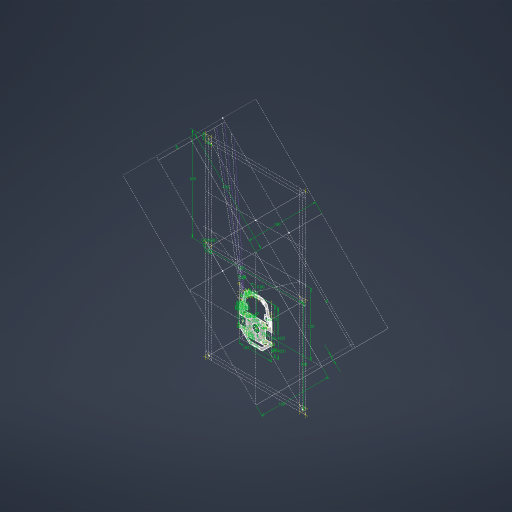
# Autodesk Inventor part: chassis
Saved by Autodesk Inventor 2023.5 (Build 275446000, 446)
## iProperties
Created: 2024-12-08
Part Number: chassis
Material: 一般
Document SubType Name: Modeling
Designer: IshiiLabHonda
Density: 1 g/cm^3
Appearance: 既定
Author: IshiiLabHonda
Autodesk Inventor part; units mm, degrees
(part 1 of 2)
ref_plane "YZ Plane" through (0, 0, 0) normal (1, 0, 0) x (0, 1, 0)
ref_plane "XZ Plane" through (0, 0, 0) normal (0, 1, 0) x (-1, 0, 0)
ref_plane "XY Plane" through (0, 0, 0) normal (0, 0, 1) x (1, 0, 0)
sketch "スケッチ1" plane through (0, 0, 0) normal (0, 0, 1) x (1, 0, 0)
  line L0 (0, 0) -> (0, 1) construction
  line L1 (0, 0) -> (1, 0) construction
  line L2 (-90, 90) -> (90, 90) construction
  line L3 (90, 90) -> (90, -90) construction
  line L4 (90, -90) -> (-90, -90) construction
  line L5 (-90, -90) -> (-90, 90) construction
  line L6 (-90, -90) -> (90, 90) construction
  line L7 (-90, 90) -> (90, -90) construction
  line L8 (-84, 96) -> (-84, 84) construction
  line L9 (-84, 84) -> (-96, 84) construction
  line L10 (-96, 84) -> (-96, 96) construction
  line L11 (-96, 96) -> (-84, 84) construction
  line L12 (-84, 96) -> (-96, 84) construction
  line L13 (-96, 96) -> (-84, 96) construction
  line L14 (-96, -96) -> (-96, -84) construction
  line L15 (-84, -96) -> (-96, -96) construction
  line L16 (-96, -96) -> (-84, -84) construction
  line L17 (-96, -84) -> (-84, -96) construction
  line L18 (-84, -84) -> (-84, -96) construction
  line L19 (-96, -84) -> (-84, -84) construction
  line L20 (96, -96) -> (84, -96) construction
  line L21 (96, -84) -> (96, -96) construction
  line L22 (96, -96) -> (84, -84) construction
  line L23 (84, -96) -> (96, -84) construction
  line L24 (84, -84) -> (96, -84) construction
  line L25 (84, -96) -> (84, -84) construction
  line L26 (96, 96) -> (96, 84) construction
  line L27 (84, 96) -> (96, 96) construction
  line L28 (96, 96) -> (84, 84) construction
  line L29 (96, 84) -> (84, 96) construction
  line L30 (84, 84) -> (84, 96) construction
  line L31 (96, 84) -> (84, 84) construction
  line L32 (-84, 84) -> (-84, -84) construction
  line L33 (-96, 84) -> (-96, -84) construction
  line L34 (-84, -84) -> (84, -84) construction
  line L35 (-84, -96) -> (84, -96) construction
  line L36 (96, 84) -> (96, -84) construction
  line L37 (84, 84) -> (84, -84) construction
  line L38 (-84, 96) -> (84, 96) construction
  line L39 (-84, 84) -> (84, 84) construction
  line L40 (-19, 15) -> (19, 15) construction
  line L41 (19, 15) -> (19, -15) construction
  line L42 (19, -15) -> (-19, -15) construction
  line L43 (-19, -15) -> (-19, 15) construction
  line L44 (-19, 15) -> (19, -15) construction
  line L45 (19, 15) -> (-19, -15) construction
  line L46 (-30.25, 11.5) -> (-19, 11.5) construction
  line L47 (-19, -11.5) -> (-30.25, -11.5) construction
  line L48 (-30.25, -11.5) -> (-30.25, 11.5) construction
  line L49 (-30.25, 11.5) -> (-19, -11.5) construction
  line L50 (-19, 11.5) -> (-30.25, -11.5) construction
  line L51 (30.25, 11.5) -> (19, 11.5) construction
  line L52 (19, -11.5) -> (30.25, -11.5) construction
  line L53 (30.25, -11.5) -> (30.25, 11.5) construction
  line L54 (30.25, 11.5) -> (19, -11.5) construction
  line L55 (19, 11.5) -> (30.25, -11.5) construction
  line L56 (-19, -10) -> (19, -10) construction
  line L57 (-19, -12.5) -> (19, -12.5) construction
  line L58 (-19, 10) -> (19, 10) construction
  line L59 (-19, 12.5) -> (19, 12.5) construction
  line L60 (-16.5, -15) -> (-16.5, 15) construction
  line L61 (16.5, -15) -> (16.5, 15) construction
  line L62 (-12.5, -10) -> (-12.5, -15) construction
  line L63 (-16.5, -10) -> (-12.5, -15) construction
  line L64 (-16.5, -15) -> (-12.5, -10) construction
  circle A0 centre (-14.5, -12.5) radius 0.8 construction
  line L65 (12.5, -10) -> (12.5, -15) construction
  line L66 (16.5, -10) -> (12.5, -15) construction
  line L67 (16.5, -15) -> (12.5, -10) construction
  circle A1 centre (14.5, -12.5) radius 0.8 construction
  line L68 (-12.5, 10) -> (-12.5, 15) construction
  line L69 (-16.5, 10) -> (-12.5, 15) construction
  line L70 (-16.5, 15) -> (-12.5, 10) construction
  circle A2 centre (-14.5, 12.5) radius 0.8 construction
  line L71 (12.5, 10) -> (12.5, 15) construction
  line L72 (16.5, 10) -> (12.5, 15) construction
  circle A3 centre (14.5, 12.5) radius 0.8 construction
  line L73 (16.5, 15) -> (12.5, 10) construction
  line L74 (-96, 276) -> (-84, 276) construction
  line L75 (-84, 276) -> (-84, 264) construction
  line L76 (-84, 264) -> (-96, 264) construction
  line L77 (-96, 264) -> (-96, 276) construction
  line L78 (-96, 276) -> (-84, 264) construction
  line L79 (-84, 276) -> (-96, 264) construction
  line L80 (-90, 90) -> (-90, 270) construction
  line L81 (-96, 264) -> (-96, 96) construction
  line L82 (-84, 264) -> (-84, 96) construction
  line L83 (96, 276) -> (84, 276) construction
  line L84 (84, 276) -> (84, 264) construction
  line L85 (84, 264) -> (96, 264) construction
  line L86 (96, 264) -> (96, 276) construction
  line L87 (96, 276) -> (84, 264) construction
  line L88 (84, 276) -> (96, 264) construction
  line L89 (90, 90) -> (90, 270) construction
  line L90 (96, 264) -> (96, 96) construction
  line L91 (84, 264) -> (84, 96) construction
  line L92 (-84, 276) -> (84, 276) construction
  line L93 (-84, 264) -> (84, 264) construction
  line L94 (-90, 270) -> (90, 270) construction
  line L95 (-90, 270) -> (90, 90) construction
  line L96 (-90, 90) -> (90, 270) construction
  circle A4 centre (0, 0) radius 15 construction
  line L97 (-96, 120) -> (96, 120) construction
  line L98 (0, 127.279221) -> (0, -127.279221) construction
  line L99 (-127.279221, 0) -> (127.279221, 0) construction
  line L100 (127.279221, 0) -> (0, -127.279221) construction
  line L101 (0, -127.279221) -> (-127.279221, 0) construction
  line L102 (-127.279221, 0) -> (0, 127.279221) construction
  line L103 (0, 127.279221) -> (127.279221, 0) construction
  line L104 (127.279221, 254.558441) -> (254.558441, 127.279221) construction
  line L105 (254.558441, 127.279221) -> (127.279221, 0) construction
  line L106 (127.279221, 0) -> (0, 127.279221) construction
  line L107 (0, 127.279221) -> (127.279221, 254.558441) construction
  line L108 (-127.279221, 254.558441) -> (0, 127.279221) construction
  line L109 (0, 127.279221) -> (-127.279221, 0) construction
  line L110 (-127.279221, 0) -> (-254.558441, 127.279221) construction
  line L111 (-254.558441, 127.279221) -> (-127.279221, 254.558441) construction
  line L112 (0, 381.837662) -> (127.279221, 254.558441) construction
  line L113 (127.279221, 254.558441) -> (0, 127.279221) construction
  line L114 (0, 127.279221) -> (-127.279221, 254.558441) construction
  line L115 (-127.279221, 254.558441) -> (0, 381.837662) construction
  line L116 (190.918831, 63.63961) -> (63.63961, 190.918831) construction
  line L117 (-190.918831, 190.918831) -> (-63.63961, 63.63961) construction
  line L118 (59.39697, -59.39697) -> (186.67619, 67.882251) construction
  line L119 (59.39697, 186.67619) -> (186.67619, 59.39697) construction
  line L120 (63.63961, 190.918831) -> (-63.63961, 318.198052) construction
  line L121 (-186.67619, 186.67619) -> (-59.39697, 313.955411) construction
  point P0 (-90, -90)
  point P1 (90, -90)
  point P2 (-24.625, 0)
  point P3 (-84, 120)
  point P4 (84, 120)
  point P5 (0, 0)
  dimension "d0" = 1
  dimension "d1" = 1
  dimension "d2" = 180
  dimension "d3" = 180
  dimension "d4" = 12
  dimension "d5" = 12
  dimension "d8" = 360
  dimension "d10" = 38
  dimension "d12" = 11.25
  dimension "d13" = 23
  dimension "d14" = 5
  dimension "d15" = 2.5
  dimension "d16" = 4
  dimension "d17" = 1.6
  dimension "d22" = 12
  dimension "d23" = 12
  dimension "d24" = 180
  dimension "d25" = 25
  dimension "d26" = 30
  dimension "d27" = 30
  dimension "d29" = 120
  dimension "d331" = 180
  dimension "d334" = 180
  dimension "d337" = 180
  dimension "d340" = 6
  dimension "d341" = 6
  dimension "d342" = 6
  dimension "d561" = 33
  constraints: 244 end point, 29 point on line, 27 symmetric about line, 19 midpoint, 18 parallel, 10 perpendicular, 5 centre point, 4 coincident, 2 collinear, 1 horizontal, 1 vertical, 91 other
  measures "d0" distance of L0.start L0.end
  measures "d1" distance of L0.start L1.end
  measures "d2" distance of L2.start L2.end
  measures "d3" distance of L2.end L3.end
  measures "d4" distance of L9.end L10.end
  measures "d5" distance of L8.end L9.end
  measures "d10" distance of L40.start L40.end
  measures "d12" distance of L46.start L46.end
  measures "d13" distance of L47.end L46.start
  measures "d14" distance between parallel lines of L56 L42
  measures "d15" distance between parallel lines of L43 L60
  measures "d16" distance between parallel lines of L60 L62
  measures "d17" diameter of A0
  measures "d22" distance of L75.end L76.end
  measures "d23" distance of L76.end L74.start
  measures "d24" distance of L2.start L80.end
  measures "d25" distance between parallel lines of L57 L59
  measures "d26" distance between parallel lines of L42 L40
  measures "d27" diameter of A4
  measures "d29" distance between parallel lines of L1 L97
  measures "d331" distance of L100.start L100.end
  measures "d334" distance of L102.end L104.start
  measures "d337" distance of L102.end L108.start
  measures "d340" distance between parallel lines of L118 L105
  measures "d341" distance between parallel lines of L116 L119
  measures "d342" distance between parallel lines of L111 L121
  measures "d561" distance between parallel lines of L61 L60
sketch "スケッチ4" plane through (0, 0, 0) normal (0, 0, 1) x (1, 0, 0)
  line L0 (-84, 264) -> (-96, 264) construction
  line L1 (-90, 90) -> (-90, 270) construction
  line L2 (-96, 264) -> (-96, 96) construction
  line L3 (-96, 96) -> (-84, 96) construction
  line L4 (-84, 96) -> (-84, 84) construction
  line L5 (-84, 96) -> (-96, 84) construction
  line L6 (-96, 96) -> (-84, 84) construction
  line L7 (-84, 264) -> (-84, 96) construction
  line L8 (-84, 84) -> (-96, 84) construction
  line L9 (84, -84) -> (96, -84) construction
  line L10 (84, -96) -> (96, -84) construction
  line L11 (96, -96) -> (84, -84) construction
  line L12 (96, -84) -> (96, -96) construction
  line L13 (96, -96) -> (84, -96) construction
  line L14 (0, 0) -> (0, 1) construction
  line L15 (0, 0) -> (1, 0) construction
  line L16 (16.5, 15) -> (12.5, 10) construction
  line L17 (-96, 84) -> (-96, -84) construction
  line L18 (-84, 84) -> (-84, -84) construction
  line L19 (-90, -90) -> (-90, 90) construction
  line L20 (-90, 90) -> (90, 90) construction
  line L21 (-84, -84) -> (84, -84) construction
  line L22 (-84, -96) -> (84, -96) construction
  line L23 (-90, -90) -> (90, 90) construction
  line L24 (90, -90) -> (-90, -90) construction
  line L25 (-90, 90) -> (90, -90) construction
  line L26 (84, 84) -> (84, -84) construction
  line L27 (90, 90) -> (90, -90) construction
  line L28 (96, 84) -> (96, -84) construction
  line L29 (-96, 84) -> (-96, 96) construction
  line L30 (-84, -84) -> (-84, -96) construction
  line L31 (-96, -84) -> (-84, -84) construction
  line L32 (-84, -96) -> (-96, -96) construction
  line L33 (-96, -96) -> (-84, -84) construction
  line L34 (-96, -84) -> (-84, -96) construction
  line L35 (-96, -96) -> (-96, -84) construction
  line L36 (84, -96) -> (84, -84) construction
  line L37 (-19, -15) -> (-19, 15) construction
  line L38 (-30.25, 11.5) -> (-19, 11.5) construction
  line L39 (-19, -11.5) -> (-30.25, -11.5) construction
  line L40 (-19, 11.5) -> (-30.25, -11.5) construction
  line L41 (-30.25, 11.5) -> (-19, -11.5) construction
  line L42 (-30.25, -11.5) -> (-30.25, 11.5) construction
  line L43 (12.5, 10) -> (12.5, 15) construction
  circle A0 centre (14.5, 12.5) radius 0.8 construction
  line L44 (30.25, 11.5) -> (19, 11.5) construction
  line L45 (16.5, 10) -> (12.5, 15) construction
  circle A1 centre (14.5, -12.5) radius 0.8 construction
  line L46 (16.5, -15) -> (12.5, -10) construction
  line L47 (16.5, -10) -> (12.5, -15) construction
  line L48 (12.5, -10) -> (12.5, -15) construction
  circle A2 centre (-14.5, -12.5) radius 0.8 construction
  line L49 (-12.5, -10) -> (-12.5, -15) construction
  line L50 (-16.5, -15) -> (-12.5, -10) construction
  line L51 (-16.5, -10) -> (-12.5, -15) construction
  line L52 (96, 84) -> (84, 84) construction
  line L53 (96, 96) -> (96, 84) construction
  line L54 (84, 96) -> (96, 96) construction
  line L55 (96, 96) -> (84, 84) construction
  line L56 (84, 84) -> (84, 96) construction
  line L57 (96, 84) -> (84, 96) construction
  line L58 (-96, 264) -> (-96, 276) construction
  line L59 (-84, 276) -> (-84, 264) construction
  line L60 (-96, 276) -> (-84, 276) construction
  line L61 (-96, 276) -> (-84, 264) construction
  line L62 (-84, 276) -> (-96, 264) construction
  line L63 (-84, 84) -> (84, 84) construction
  line L64 (-84, 96) -> (84, 96) construction
  line L65 (84, 264) -> (84, 96) construction
  line L66 (90, 90) -> (90, 270) construction
  line L67 (-90, 90) -> (90, 270) construction
  line L68 (-90, 270) -> (90, 90) construction
  line L69 (96, 264) -> (96, 96) construction
  line L70 (-96, 120) -> (96, 120) construction
  line L71 (-84, 264) -> (84, 264) construction
  line L72 (-84, 276) -> (84, 276) construction
  line L73 (-90, 270) -> (90, 270) construction
  line L74 (84, 276) -> (84, 264) construction
  line L75 (84, 264) -> (96, 264) construction
  line L76 (96, 264) -> (96, 276) construction
  line L77 (96, 276) -> (84, 264) construction
  line L78 (96, 276) -> (84, 276) construction
  line L79 (84, 276) -> (96, 264) construction
  line L80 (-19, 15) -> (19, 15) construction
  line L81 (19, 15) -> (19, -15) construction
  line L82 (19, -15) -> (-19, -15) construction
  circle A3 centre (-14.5, 12.5) radius 0.8 construction
  line L83 (-16.5, 10) -> (-12.5, 15) construction
  line L84 (-12.5, 10) -> (-12.5, 15) construction
  line L85 (-16.5, 15) -> (-12.5, 10) construction
  circle A4 centre (0, 0) radius 15 construction
  line L86 (-19, 10) -> (19, 10) construction
  line L87 (-19, 12.5) -> (19, 12.5) construction
  line L88 (-19, 15) -> (19, -15) construction
  line L89 (19, 15) -> (-19, -15) construction
  line L90 (-19, -10) -> (19, -10) construction
  line L91 (-19, -12.5) -> (19, -12.5) construction
  line L92 (16.5, -15) -> (16.5, 15) construction
  line L93 (19, 11.5) -> (30.25, -11.5) construction
  line L94 (19, -11.5) -> (30.25, -11.5) construction
  line L95 (30.25, -11.5) -> (30.25, 11.5) construction
  line L96 (30.25, 11.5) -> (19, -11.5) construction
  line L97 (-16.5, -15) -> (-16.5, 15) construction
  line L98 (-84, 120) -> (30.25, 40.001289) construction
  line L99 (84, 120) -> (-30.25, 40.001289) construction
  line L100 (-30.25, 57) -> (30.25, 57) construction
  line L101 (1.000463, 57) -> (-30.25, 35.11819) construction
  line L102 (-1.000463, 57) -> (30.25, 35.11819) construction
  line L103 (-12.947112, 57) -> (-30.25, 44.884387) construction
  line L104 (-14.32927, 55.421815) -> (-10.314235, 49.68775) construction
  line L105 (-10.314235, 49.68775) -> (-15.638724, 45.959504) construction
  line L106 (-15.638724, 45.959504) -> (-19.653759, 51.693568) construction
  line L107 (-19.653759, 51.693568) -> (-14.32927, 55.421815) construction
  line L108 (-14.32927, 55.421815) -> (-15.638724, 45.959504) construction
  line L109 (-10.314235, 49.68775) -> (-19.653759, 51.693568) construction
  line L110 (-13.755694, 54.602663) -> (-19.080182, 50.874416) construction
  line L111 (-10.887812, 50.506903) -> (-16.2123, 46.778656) construction
  line L112 (-14.983997, 50.690659) -> (-14.328675, 51.14952) construction
  line L113 (-14.983997, 50.690659) -> (-14.525136, 50.035338) construction
  line L114 (-14.615634, 52.779752) -> (-12.894904, 50.322296) construction
  line L115 (-12.894904, 50.322296) -> (-15.35236, 48.601566) construction
  line L116 (-15.35236, 48.601566) -> (-17.07309, 51.059023) construction
  line L117 (-17.07309, 51.059023) -> (-14.615634, 52.779752) construction
  line L118 (-14.615634, 52.779752) -> (-15.35236, 48.601566) construction
  line L119 (-12.894904, 50.322296) -> (-17.07309, 51.059023) construction
  circle A5 centre (-14.983997, 50.690659) radius 0.8 construction
  line L120 (-30.25, 11.5) -> (-30.25, 57) construction
  line L121 (30.25, 11.5) -> (30.25, 57) construction
  line L122 (-6.140277, 52) -> (6.140277, 52) construction
  line L123 (-31, 57) -> (-31, -31) construction
  line L124 (31, 57) -> (31, -31) construction
  line L125 (-30.25, 57) -> (-31, 57) construction
  line L126 (30.25, 57) -> (31, 57) construction
  line L127 (-31, 8.5) -> (31, 8.5) construction
  line L128 (-31, -8.5) -> (31, -8.5) construction
  circle A6 centre (0, 0) radius 7.5 construction
  line L129 (-31, -31) -> (31, -31) construction
  line L130 (-30.25, 44.884387) -> (-31, 44.359231) construction
  line L131 (-30.25, 35.11819) -> (-31, 34.593035) construction
  line L132 (-25.25, 26.5) -> (-25.361338, 27.292214) construction
  line L133 (-25.25, 26.5) -> (-24.457786, 26.611338) construction
  line L134 (-28.073603, 28.627737) -> (-23.122263, 29.323603) construction
  line L135 (-23.122263, 29.323603) -> (-22.426397, 24.372263) construction
  line L136 (-22.426397, 24.372263) -> (-27.377737, 23.676397) construction
  line L137 (-27.377737, 23.676397) -> (-28.073603, 28.627737) construction
  line L138 (-28.073603, 28.627737) -> (-22.426397, 24.372263) construction
  line L139 (-23.122263, 29.323603) -> (-27.377737, 23.676397) construction
  circle A7 centre (-25.25, 26.5) radius 0.8 construction
  line L140 (-25.25, 57) -> (-25.25, -31) construction
  line L141 (-96, 180) -> (96, 180) construction
  line L142 (-25.361338, 27.292214) -> (-64.878802, 308.473578) construction
  line L143 (-186.67619, 186.67619) -> (-59.39697, 313.955411) construction
  line L144 (59.39697, 186.67619) -> (186.67619, 59.39697) construction
  line L145 (-25.25, 26.5) -> (-79.619204, 293.733176) construction
  line L146 (-25.25, 26.5) -> (-46.888819, 301.44726) construction
  line L147 (63.63961, 190.918831) -> (-63.63961, 318.198052) construction
  line L148 (14.32927, 55.421815) -> (10.314235, 49.68775) construction
  line L149 (10.314235, 49.68775) -> (15.638724, 45.959504) construction
  line L150 (15.638724, 45.959504) -> (19.653759, 51.693568) construction
  line L151 (19.653759, 51.693568) -> (14.32927, 55.421815) construction
  line L152 (14.32927, 55.421815) -> (15.638724, 45.959504) construction
  line L153 (10.314235, 49.68775) -> (19.653759, 51.693568) construction
  line L154 (13.755694, 54.602663) -> (19.080182, 50.874416) construction
  line L155 (10.887812, 50.506903) -> (16.2123, 46.778656) construction
  line L156 (14.983997, 50.690659) -> (14.328675, 51.14952) construction
  line L157 (14.983997, 50.690659) -> (14.525136, 50.035338) construction
  line L158 (14.615634, 52.779752) -> (12.894904, 50.322296) construction
  line L159 (12.894904, 50.322296) -> (15.35236, 48.601566) construction
  line L160 (15.35236, 48.601566) -> (17.07309, 51.059023) construction
  line L161 (17.07309, 51.059023) -> (14.615634, 52.779752) construction
  line L162 (14.615634, 52.779752) -> (15.35236, 48.601566) construction
  line L163 (12.894904, 50.322296) -> (17.07309, 51.059023) construction
  circle A8 centre (14.983997, 50.690659) radius 0.8 construction
  line L164 (-23.122263, 29.323603) -> (-18.170922, 30.019468) construction
  line L165 (-18.170922, 30.019468) -> (-17.475057, 25.068128) construction
  line L166 (-17.475057, 25.068128) -> (-22.426397, 24.372263) construction
  line L167 (-23.122263, 29.323603) -> (-28.073603, 28.627737) construction
  line L168 (-28.073603, 28.627737) -> (-27.377737, 23.676397) construction
  line L169 (-27.377737, 23.676397) -> (-22.426397, 24.372263) construction
  line L170 (27.377737, 23.676397) -> (28.073603, 28.627737) construction
  line L171 (23.122263, 29.323603) -> (18.170922, 30.019468) construction
  line L172 (18.170922, 30.019468) -> (17.475057, 25.068128) construction
  line L173 (17.475057, 25.068128) -> (22.426397, 24.372263) construction
  line L174 (23.122263, 29.323603) -> (28.073603, 28.627737) construction
  line L175 (28.073603, 28.627737) -> (27.377737, 23.676397) construction
  line L176 (27.377737, 23.676397) -> (22.426397, 24.372263) construction
  line L177 (23.122263, 29.323603) -> (27.377737, 23.676397) construction
  line L178 (22.426397, 24.372263) -> (28.073603, 28.627737) construction
  line L179 (-20.29866, 27.195866) -> (-60.451834, 312.900546) construction
  line L180 (-20.29866, 27.195866) -> (-75.387283, 297.965098) construction
  line L181 (-20.29866, 27.195866) -> (-41.455067, 296.013508) construction
  line L182 (-23.122263, 29.323603) -> (-17.475057, 25.068128) construction
  line L183 (-22.426397, 24.372263) -> (-18.170922, 30.019468) construction
  line L184 (-19.653759, 51.693568) -> (-22.111215, 49.972839) construction
  line L185 (-22.111215, 49.972839) -> (-18.09618, 44.238774) construction
  line L186 (-18.09618, 44.238774) -> (-15.638724, 45.959504) construction
  point P0 (90, -90)
  point P1 (-90, -90)
  point P2 (-24.625, 0)
  point P3 (0, 61.182567)
  point P4 (-5.973324, 57)
  point P5 (-12.321753, 52.554783)
  point P6 (0, 180)
  point P7 (12.321753, 52.554783)
  dimension "d264" = 110
  dimension "d275" = 7
  dimension "d276" = 6.5
  dimension "d277" = 5
  dimension "d278" = 3
  dimension "d279" = 3
  dimension "d280" = 1.6
  dimension "d281" = 8
  dimension "d284" = 5
  dimension "d288" = 17
  dimension "d289" = 15
  dimension "d290" = 0.75
  dimension "d291" = 0.75
  dimension "d292" = 88
  dimension "d296" = 5
  dimension "d297" = 5
  dimension "d298" = 1.6
  dimension "d299" = 8
  dimension "d345" = 7
  dimension "d346" = 15
  dimension "d356" = 16
  dimension "d367" = 5
  dimension "d369" = 42
  dimension "d370" = 11
  dimension "d371" = 62
  dimension "d382" = 5
  dimension "d385" = 7
  dimension "d513" = 3
  constraints: 172 end point, 38 point on line, 25 symmetric about line, 19 parallel, 15 perpendicular, 13 midpoint, 6 point on circle, 5 collinear, 4 centre point, 4 coincident, 2 equal length, 8 other
  measures "d264" angle of L99 L98
  measures "d275" distance of L104.start L104.end
  measures "d276" distance of L106.end L104.start
  measures "d277" distance between parallel lines of L110 L111
  measures "d278" distance of L115.end L116.end
  measures "d279" distance of L114.end L115.end
  measures "d280" diameter of A5
  measures "d281" distance between parallel lines of L101 L103
  measures "d284" distance between parallel lines of L100 L122
  measures "d288" distance between parallel lines of L128 L127
  measures "d289" diameter of A6
  measures "d290" distance between parallel lines of L123 L120
  measures "d291" distance between parallel lines of L121 L124
  measures "d292" distance between parallel lines of L129 L100
  measures "d296" distance of L135.end L136.end
  measures "d297" distance of L134.end L135.end
  measures "d298" diameter of A7
  measures "d299" angle of L140 L132
  measures "d345" angle of L145 L146
  measures "d346" distance from line of L38 L132.start
  measures "d356" distance between parallel lines of L129 L82
  measures "d367" distance between parallel lines of L120 L140
  measures "d369" distance between parallel lines of L80 L100
  measures "d370" distance of L112.start point (-5.973, 57)
  measures "d371" distance of L123.end L124.end
  measures "d382" distance of L134.end L164.end
  measures "d385" angle of L180 L181
  measures "d513" distance between parallel lines of L185 L106
sketch "スケッチ5" plane through (0, 0, 0) normal (0, 0, 1) x (1, 0, 0)
  line L0 (0, 0) -> (0, 1) construction
  line L1 (30.25, 11.5) -> (19, 11.5) construction
  line L2 (19, 11.5) -> (30.25, -11.5) construction
  line L3 (30.25, 11.5) -> (19, -11.5) construction
  line L4 (30.25, -11.5) -> (30.25, 11.5) construction
  line L5 (19, -11.5) -> (30.25, -11.5) construction
  line L6 (-90, 90) -> (90, 90) construction
  line L7 (-90, -90) -> (90, 90) construction
  line L8 (-90, 90) -> (90, -90) construction
  line L9 (-84, 84) -> (-84, -84) construction
  line L10 (-96, 84) -> (-96, -84) construction
  line L11 (-90, -90) -> (-90, 90) construction
  line L12 (-84, 84) -> (-96, 84) construction
  line L13 (-96, 84) -> (-96, 96) construction
  line L14 (84, 84) -> (84, -84) construction
  line L15 (90, 90) -> (90, -90) construction
  line L16 (96, 84) -> (84, 84) construction
  line L17 (96, 84) -> (96, -84) construction
  line L18 (90, -90) -> (-90, -90) construction
  line L19 (-84, -84) -> (84, -84) construction
  line L20 (-84, -96) -> (84, -96) construction
  line L21 (-84, -84) -> (-84, -96) construction
  line L22 (-96, -96) -> (-96, -84) construction
  line L23 (-84, -96) -> (-96, -96) construction
  line L24 (-96, -96) -> (-84, -84) construction
  line L25 (-96, -84) -> (-84, -96) construction
  line L26 (-96, -84) -> (-84, -84) construction
  line L27 (0, 0) -> (1, 0) construction
  line L28 (-84, 264) -> (-96, 264) construction
  line L29 (-96, 276) -> (-84, 276) construction
  line L30 (-96, 264) -> (-96, 276) construction
  line L31 (-84, 276) -> (-96, 264) construction
  line L32 (-96, 276) -> (-84, 264) construction
  line L33 (-84, 276) -> (-84, 264) construction
  line L34 (84, -96) -> (84, -84) construction
  line L35 (96, -96) -> (84, -96) construction
  line L36 (96, -84) -> (96, -96) construction
  line L37 (96, -96) -> (84, -84) construction
  line L38 (84, -96) -> (96, -84) construction
  line L39 (84, -84) -> (96, -84) construction
  line L40 (-19, 15) -> (19, 15) construction
  line L41 (19, 15) -> (19, -15) construction
  line L42 (16.5, 15) -> (12.5, 10) construction
  line L43 (12.5, 10) -> (12.5, 15) construction
  line L44 (16.5, 10) -> (12.5, 15) construction
  line L45 (16.5, -15) -> (16.5, 15) construction
  line L46 (-19, 10) -> (19, 10) construction
  line L47 (-19, 12.5) -> (19, 12.5) construction
  circle A0 centre (0, 0) radius 15 construction
  line L48 (-19, -10) -> (19, -10) construction
  line L49 (-19, -12.5) -> (19, -12.5) construction
  line L50 (19, -15) -> (-19, -15) construction
  line L51 (-19, 15) -> (19, -15) construction
  line L52 (19, 15) -> (-19, -15) construction
  line L53 (-16.5, -15) -> (-16.5, 15) construction
  line L54 (-19, -15) -> (-19, 15) construction
  line L55 (-30.25, 11.5) -> (-19, 11.5) construction
  line L56 (-19, -11.5) -> (-30.25, -11.5) construction
  line L57 (-30.25, -11.5) -> (-30.25, 11.5) construction
  line L58 (-30.25, 11.5) -> (-19, -11.5) construction
  line L59 (-19, 11.5) -> (-30.25, -11.5) construction
  line L60 (-12.5, 10) -> (-12.5, 15) construction
  circle A1 centre (-14.5, 12.5) radius 0.8 construction
  line L61 (-16.5, 10) -> (-12.5, 15) construction
  line L62 (-16.5, 15) -> (-12.5, 10) construction
  circle A2 centre (14.5, 12.5) radius 0.8 construction
  line L63 (-84, 96) -> (-96, 84) construction
  line L64 (-96, 96) -> (-84, 96) construction
  line L65 (-84, 96) -> (-84, 84) construction
  line L66 (-96, 96) -> (-84, 84) construction
  line L67 (-96, 264) -> (-96, 96) construction
  line L68 (-84, 264) -> (-84, 96) construction
  line L69 (-84, 96) -> (84, 96) construction
  line L70 (-84, 84) -> (84, 84) construction
  line L71 (84, 84) -> (84, 96) construction
  line L72 (96, 96) -> (96, 84) construction
  line L73 (96, 96) -> (84, 84) construction
  line L74 (96, 84) -> (84, 96) construction
  line L75 (-96, 120) -> (96, 120) construction
  line L76 (84, 96) -> (96, 96) construction
  line L77 (-84, 264) -> (84, 264) construction
  line L78 (84, 264) -> (84, 96) construction
  line L79 (-84, 276) -> (84, 276) construction
  line L80 (96, 264) -> (96, 96) construction
  line L81 (-90, 270) -> (90, 270) construction
  line L82 (-90, 270) -> (90, 90) construction
  line L83 (-90, 90) -> (90, 270) construction
  line L84 (90, 90) -> (90, 270) construction
  line L85 (-90, 90) -> (-90, 270) construction
  line L86 (84, 264) -> (96, 264) construction
  line L87 (96, 276) -> (84, 276) construction
  line L88 (96, 276) -> (84, 264) construction
  line L89 (84, 276) -> (96, 264) construction
  line L90 (96, 264) -> (96, 276) construction
  line L91 (84, 276) -> (84, 264) construction
  circle A3 centre (-14.5, -12.5) radius 0.8 construction
  line L92 (-12.5, -10) -> (-12.5, -15) construction
  line L93 (-16.5, -15) -> (-12.5, -10) construction
  line L94 (12.5, -10) -> (12.5, -15) construction
  circle A4 centre (14.5, -12.5) radius 0.8 construction
  line L95 (16.5, -15) -> (12.5, -10) construction
  line L96 (16.5, -10) -> (12.5, -15) construction
  line L97 (-16.5, -10) -> (-12.5, -15) construction
  line L98 (-17.07309, 51.059023) -> (-14.615634, 52.779752) construction
  line L99 (-12.894904, 50.322296) -> (-17.07309, 51.059023) construction
  circle A5 centre (-14.983997, 50.690659) radius 0.8 construction
  line L100 (-12.894904, 50.322296) -> (-15.35236, 48.601566) construction
  line L101 (-14.615634, 52.779752) -> (-15.35236, 48.601566) construction
  line L102 (-15.35236, 48.601566) -> (-17.07309, 51.059023) construction
  line L103 (-30.25, 44.884387) -> (-31, 44.359231) construction
  line L104 (-12.947112, 57) -> (-30.25, 44.884387) construction
  line L105 (-30.25, 57) -> (-31, 57) construction
  line L106 (-14.615634, 52.779752) -> (-12.894904, 50.322296) construction
  line L107 (-30.25, 57) -> (30.25, 57) construction
  line L108 (-10.314235, 49.68775) -> (-15.638724, 45.959504) construction
  line L109 (-15.638724, 45.959504) -> (-19.653759, 51.693568) construction
  line L110 (-14.32927, 55.421815) -> (-10.314235, 49.68775) construction
  line L111 (1.000463, 57) -> (-30.25, 35.11819) construction
  line L112 (-1.000463, 57) -> (30.25, 35.11819) construction
  line L113 (-19, 15) -> (19, 15) construction
  line L114 (12.5, 10) -> (12.5, 15) construction
  line L115 (-19, 10) -> (19, 10) construction
  circle A6 centre (-14.5, 12.5) radius 0.8 construction
  line L116 (-12.5, 10) -> (-12.5, 15) construction
  line L117 (-16.5, 10) -> (-12.5, 15) construction
  line L118 (-16.5, 15) -> (-12.5, 10) construction
  line L119 (-19, 12.5) -> (19, 12.5) construction
  line L120 (30.25, 57) -> (31, 57) construction
  line L121 (30.25, 11.5) -> (30.25, 57) construction
  line L122 (-6.140277, 52) -> (6.140277, 52) construction
  line L123 (-30.25, 35.11819) -> (-31, 34.593035) construction
  line L124 (-30.25, 11.5) -> (-30.25, 57) construction
  line L125 (-10.887812, 50.506903) -> (-16.2123, 46.778656) construction
  line L126 (-14.983997, 50.690659) -> (-14.525136, 50.035338) construction
  line L127 (-14.983997, 50.690659) -> (-14.328675, 51.14952) construction
  line L128 (-10.314235, 49.68775) -> (-19.653759, 51.693568) construction
  line L129 (-13.755694, 54.602663) -> (-19.080182, 50.874416) construction
  line L130 (-19.653759, 51.693568) -> (-14.32927, 55.421815) construction
  line L131 (-14.32927, 55.421815) -> (-15.638724, 45.959504) construction
  line L132 (-30.25, 11.5) -> (-19, 11.5) construction
  line L133 (-30.25, 11.5) -> (-19, -11.5) construction
  line L134 (30.25, 11.5) -> (19, 11.5) construction
  line L135 (30.25, -11.5) -> (30.25, 11.5) construction
  line L136 (19, 11.5) -> (30.25, -11.5) construction
  line L137 (30.25, 11.5) -> (19, -11.5) construction
  line L138 (0, 0) -> (0, 1) construction
  line L139 (0, 0) -> (1, 0) construction
  circle A7 centre (0, 0) radius 7.5 construction
  circle A8 centre (0, 0) radius 15 construction
  line L140 (-16.5, -15) -> (-16.5, 15) construction
  circle A9 centre (14.5, 12.5) radius 0.8 construction
  line L141 (-12.5, -10) -> (-12.5, -15) construction
  line L142 (12.5, -10) -> (12.5, -15) construction
  line L143 (16.5, 10) -> (12.5, 15) construction
  line L144 (-16.5, -15) -> (-12.5, -10) construction
  line L145 (16.5, -10) -> (12.5, -15) construction
  line L146 (16.5, 15) -> (12.5, 10) construction
  line L147 (-19, -12.5) -> (19, -12.5) construction
  line L148 (19, -15) -> (-19, -15) construction
  line L149 (-19, 11.5) -> (-30.25, -11.5) construction
  line L150 (19, -11.5) -> (30.25, -11.5) construction
  line L151 (-19, -11.5) -> (-30.25, -11.5) construction
  line L152 (-30.25, -11.5) -> (-30.25, 11.5) construction
  line L153 (16.5, -15) -> (16.5, 15) construction
  line L154 (19, 15) -> (19, -15) construction
  line L155 (-19, -15) -> (-19, 15) construction
  line L156 (-19, 15) -> (19, -15) construction
  line L157 (19, 15) -> (-19, -15) construction
  line L158 (-31, -8.5) -> (31, -8.5) construction
  line L159 (-31, 8.5) -> (31, 8.5) construction
  line L160 (-31, -31) -> (31, -31) construction
  line L161 (-31, 57) -> (-31, -31) construction
  line L162 (31, 57) -> (31, -31) construction
  line L163 (84, -84) -> (96, -84) construction
  line L164 (84, -96) -> (96, -84) construction
  line L165 (96, -96) -> (84, -84) construction
  line L166 (96, -84) -> (96, -96) construction
  line L167 (96, -96) -> (84, -96) construction
  line L168 (-96, 84) -> (-96, -84) construction
  line L169 (-84, 84) -> (-84, -84) construction
  line L170 (-90, -90) -> (-90, 90) construction
  line L171 (-84, -84) -> (84, -84) construction
  line L172 (-84, -96) -> (84, -96) construction
  line L173 (-90, -90) -> (90, 90) construction
  line L174 (90, -90) -> (-90, -90) construction
  line L175 (-90, 90) -> (90, -90) construction
  line L176 (84, 84) -> (84, -84) construction
  line L177 (90, 90) -> (90, -90) construction
  line L178 (96, 84) -> (96, -84) construction
  line L179 (84, -96) -> (84, -84) construction
  line L180 (-19, -10) -> (19, -10) construction
  circle A10 centre (14.5, -12.5) radius 0.8 construction
  line L181 (16.5, -15) -> (12.5, -10) construction
  line L182 (-16.5, -10) -> (-12.5, -15) construction
  line L183 (-84, -84) -> (-84, -96) construction
  line L184 (-96, -84) -> (-84, -84) construction
  line L185 (-84, -96) -> (-96, -96) construction
  line L186 (-96, -96) -> (-84, -84) construction
  line L187 (-96, -84) -> (-84, -96) construction
  line L188 (-96, -96) -> (-96, -84) construction
  circle A11 centre (-14.5, -12.5) radius 0.8 construction
  line L189 (-96, 96) -> (-84, 96) construction
  line L190 (-84, 96) -> (-84, 84) construction
  line L191 (-84, 96) -> (-96, 84) construction
  line L192 (-96, 96) -> (-84, 84) construction
  line L193 (84, 96) -> (96, 96) construction
  line L194 (96, 84) -> (84, 84) construction
  line L195 (96, 96) -> (96, 84) construction
  line L196 (96, 96) -> (84, 84) construction
  line L197 (96, 84) -> (84, 96) construction
  line L198 (-96, 120) -> (96, 120) construction
  line L199 (-84, 96) -> (84, 96) construction
  line L200 (-90, 90) -> (90, 90) construction
  line L201 (-84, 84) -> (-96, 84) construction
  line L202 (-96, 84) -> (-96, 96) construction
  line L203 (-84, 84) -> (84, 84) construction
  line L204 (84, 120) -> (-30.25, 40.001289) construction
  line L205 (-84, 120) -> (30.25, 40.001289) construction
  line L206 (84, 84) -> (84, 96) construction
  line L207 (-84, 264) -> (-96, 264) construction
  line L208 (-90, 90) -> (-90, 270) construction
  line L209 (-96, 264) -> (-96, 96) construction
  line L210 (-84, 264) -> (-84, 96) construction
  line L211 (96, 264) -> (96, 96) construction
  line L212 (84, 264) -> (84, 96) construction
  line L213 (90, 90) -> (90, 270) construction
  line L214 (-90, 90) -> (90, 270) construction
  line L215 (-90, 270) -> (90, 90) construction
  line L216 (-84, 264) -> (84, 264) construction
  line L217 (-90, 270) -> (90, 270) construction
  line L218 (-96, 264) -> (-96, 276) construction
  line L219 (-96, 276) -> (-84, 276) construction
  line L220 (-96, 276) -> (-84, 264) construction
  line L221 (-84, 276) -> (-96, 264) construction
  line L222 (-84, 276) -> (-84, 264) construction
  line L223 (-84, 276) -> (84, 276) construction
  line L224 (84, 264) -> (96, 264) construction
  line L225 (96, 264) -> (96, 276) construction
  line L226 (96, 276) -> (84, 264) construction
  line L227 (96, 276) -> (84, 276) construction
  line L228 (84, 276) -> (96, 264) construction
  line L229 (84, 276) -> (84, 264) construction
  line L230 (-31, 8.5) -> (-19, 8.5)
  line L231 (-31, -8.5) -> (-19, -8.5)
  line L232 (-19, 8.5) -> (-19, -8.5)
  circle A12 centre (0, 0) radius 7.5
  line L233 (31, 8.5) -> (19, 8.5)
  line L234 (31, -8.5) -> (19, -8.5)
  line L235 (19, 8.5) -> (19, -8.5)
  line L236 (31, 8.5) -> (31, 8.5)
  line L237 (-31, -8.5) -> (-12.120258, -31) construction
  line L238 (-12.120258, -31) -> (12.120258, -31)
  line L239 (31, -8.5) -> (12.120258, -31) construction
  circle A13 centre (-14.5, 12.5) radius 1.05
  circle A14 centre (14.5, 12.5) radius 1.05
  circle A15 centre (-14.5, -12.5) radius 1.05
  circle A16 centre (14.5, -12.5) radius 1.05
  line L240 (-25.25, 26.5) -> (-25.361338, 27.292214) construction
  line L241 (-25.25, 26.5) -> (-24.457786, 26.611338) construction
  circle A17 centre (-25.25, 26.5) radius 0.8 construction
  line L242 (-23.122263, 29.323603) -> (-22.426397, 24.372263) construction
  line L243 (-27.377737, 23.676397) -> (-28.073603, 28.627737) construction
  line L244 (-23.122263, 29.323603) -> (-27.377737, 23.676397) construction
  line L245 (-28.073603, 28.627737) -> (-23.122263, 29.323603) construction
  line L246 (-22.426397, 24.372263) -> (-27.377737, 23.676397) construction
  line L247 (-28.073603, 28.627737) -> (-22.426397, 24.372263) construction
  line L248 (-28.073603, 28.627737) -> (-27.377737, 23.676397)
  line L249 (-23.122263, 29.323603) -> (-18.170922, 30.019468) construction
  line L250 (-18.170922, 30.019468) -> (-17.475057, 25.068128) construction
  line L251 (-17.475057, 25.068128) -> (-22.426397, 24.372263) construction
  line L252 (27.377737, 23.676397) -> (22.426397, 24.372263) construction
  line L253 (17.475057, 25.068128) -> (22.426397, 24.372263) construction
  line L254 (18.170922, 30.019468) -> (17.475057, 25.068128) construction
  line L255 (23.122263, 29.323603) -> (18.170922, 30.019468) construction
  line L256 (23.122263, 29.323603) -> (28.073603, 28.627737) construction
  line L257 (28.073603, 28.627737) -> (27.377737, 23.676397) construction
  line L258 (-28.073603, 28.627737) -> (-18.170922, 30.019468)
  line L259 (-17.475057, 25.068128) -> (-18.170922, 30.019468)
  line L260 (-17.475057, 25.068128) -> (-27.377737, 23.676397)
  line L261 (18.170922, 30.019468) -> (28.073603, 28.627737)
  line L262 (27.377737, 23.676397) -> (28.073603, 28.627737)
  line L263 (27.377737, 23.676397) -> (17.475057, 25.068128)
  line L264 (18.170922, 30.019468) -> (17.475057, 25.068128)
  line L265 (-13.772846, 56.421815) -> (13.772846, 56.421815)
  line L266 (-13.772846, 56.421815) -> (-13.772846, 56.421815)
  line L267 (-7.772846, 56.421815) -> (-5.025368, 55.421815)
  line L268 (-5.025368, 55.421815) -> (5.025368, 55.421815)
  line L269 (5.025368, 55.421815) -> (7.772846, 56.421815)
  line L270 (-8.709458, 51.421815) -> (8.709458, 51.421815)
  line L271 (-18.173561, 44.794978) -> (-8.709458, 51.421815)
  line L272 (-31, 8.5) -> (-22.045093, 50.629525)
  line L273 (-22.045093, 50.629525) -> (-13.772846, 56.421815)
  line L274 (31, 8.5) -> (22.045093, 50.629525)
  line L275 (-18.173561, 44.794978) -> (-23.656453, 19)
  line L276 (18.173561, 44.794978) -> (23.656453, 19)
  line L277 (-23.656453, 19) -> (23.656453, 19)
  line L278 (-17.630844, -20) -> (17.630844, -20)
  line L279 (17.630844, -20) -> (11.507684, -26)
  line L280 (11.507684, -26) -> (-11.507684, -26)
  line L281 (-11.507684, -26) -> (-17.630844, -20)
  line L282 (-31, -8.5) -> (-31, -12.5)
  line L283 (-31, -12.5) -> (-12.120258, -31)
  line L284 (31, -8.5) -> (31, -12.5)
  line L285 (31, -12.5) -> (12.120258, -31)
  line L286 (-31, 8.5) -> (-31, 26.5)
  line L287 (-31, 26.5) -> (-26.343459, 30.407302)
  line L288 (31, 8.5) -> (31, 26.5)
  line L289 (31, 26.5) -> (26.343459, 30.407302)
  line L290 (-8.120258, -31) -> (-6.620258, -29.5)
  line L291 (-6.620258, -29.5) -> (6.620258, -29.5)
  line L292 (6.620258, -29.5) -> (8.120258, -31)
  line L293 (18.173561, 44.794978) -> (8.709458, 51.421815)
  line L294 (22.045093, 50.629525) -> (13.772846, 56.421815)
  line L295 (-23.656453, 19) -> (-24.825514, 13.5)
  line L296 (-24.825514, 13.5) -> (-20.825514, 13.5)
  line L297 (-20.825514, 13.5) -> (-15.325514, 19)
  line L298 (23.656453, 19) -> (24.825514, 13.5)
  line L299 (24.825514, 13.5) -> (20.825514, 13.5)
  line L300 (20.825514, 13.5) -> (15.325514, 19)
  line L301 (-17.630844, -20) -> (-24.264266, -13.5)
  line L302 (-24.264266, -13.5) -> (-21.264266, -13.5)
  line L303 (-21.264266, -13.5) -> (-11.630844, -20)
  line L304 (17.630844, -20) -> (24.264266, -13.5)
  line L305 (24.264266, -13.5) -> (21.264266, -13.5)
  line L306 (21.264266, -13.5) -> (11.630844, -20)
  circle A18 centre (-10.130844, -17) radius 0.625 construction
  circle A19 centre (-10.130844, -17) radius 0.8
  circle A20 centre (-10.130844, -17) radius 1.5
  line L307 (-11.630844, -20) -> (-11.630844, -15) construction
  circle A21 centre (10.130844, -17) radius 0.625 construction
  circle A22 centre (10.130844, -17) radius 0.8
  circle A23 centre (10.130844, -17) radius 1.5
  circle A24 centre (-9, 15.5) radius 0.625 construction
  circle A25 centre (-9, 15.5) radius 0.8
  circle A26 centre (-9, 15.5) radius 1.5
  circle A27 centre (9, 15.5) radius 0.625 construction
  circle A28 centre (9, 15.5) radius 0.8
  circle A29 centre (9, 15.5) radius 1.5
  circle A30 centre (-21.034754, 43.358463) radius 0.8
  circle A31 centre (-21.034754, 43.358463) radius 1.5 construction
  circle A32 centre (21.034754, 43.358463) radius 0.475 construction
  circle A33 centre (21.034754, 43.358463) radius 0.8
  circle A34 centre (21.034754, 43.358463) radius 1.5 construction
  line L308 (-29.872145, 30.647081) -> (-16.99866, 32.456331)
  line L309 (-16.99866, 32.456331) -> (-15.676515, 23.048785)
  line L310 (-15.676515, 23.048785) -> (-28.55, 21.239534)
  line L311 (-28.55, 21.239534) -> (-29.872145, 30.647081)
  line L312 (-22.045093, 50.629525) -> (-18.173561, 44.794978) construction
  line L313 (-21.81067, 27.683727) -> (-26, 24.168462)
  line L314 (-26, 24.168462) -> (-26, 13.5)
  line L315 (-24.825514, 13.5) -> (-26, 13.5)
  line L316 (21.81067, 27.683727) -> (26, 24.168462)
  line L317 (26, 24.168462) -> (26, 13.5)
  line L318 (24.825514, 13.5) -> (26, 13.5)
  circle A35 centre (-28.5, 18.5) radius 0.475 construction
  circle A36 centre (-28.5, 18.5) radius 0.8
  circle A37 centre (-28.5, 18.5) radius 1.5
  circle A38 centre (28.5, 18.5) radius 0.8
  circle A39 centre (28.5, 18.5) radius 1.5
  circle A40 centre (28.5, 18.5) radius 0.475 construction
  line L319 (-12.947112, 57) -> (12.947112, 57)
  line L320 (29.872145, 30.647081) -> (16.99866, 32.456331)
  line L321 (16.99866, 32.456331) -> (15.676515, 23.048785)
  line L322 (15.676515, 23.048785) -> (28.55, 21.239534)
  line L323 (28.55, 21.239534) -> (29.872145, 30.647081)
  line L324 (-23.480123, 43.878242) -> (-18.589385, 42.838683) construction
  line L325 (-20.109327, 47.712252) -> (-28.444149, 8.5) construction
  line L326 (-17.351635, 51.108138) -> (-14.566518, 53.058298)
  line L327 (-14.566518, 53.058298) -> (-12.616358, 50.273181)
  line L328 (-12.616358, 50.273181) -> (-15.401475, 48.323021)
  line L329 (-15.401475, 48.323021) -> (-17.351635, 51.108138)
  line L330 (-17.351635, 51.108138) -> (-12.616358, 50.273181) construction
  line L331 (-14.566518, 53.058298) -> (-15.401475, 48.323021) construction
  line L332 (17.351635, 51.108138) -> (14.566518, 53.058298)
  line L333 (14.566518, 53.058298) -> (12.616358, 50.273181)
  line L334 (12.616358, 50.273181) -> (15.401475, 48.323021)
  line L335 (15.401475, 48.323021) -> (17.351635, 51.108138)
  circle A41 centre (-14.983997, 50.690659) radius 1.05
  circle A42 centre (14.983997, 50.690659) radius 1.05
  point P0 (-90, -90)
  point P1 (90, -90)
  point P2 (-24.625, 0)
  point P3 (-12.321753, 52.554783)
  point P4 (-5.973324, 57)
  point P5 (0, 61.182567)
  point P6 (-24.625, 0)
  point P7 (-90, -90)
  point P8 (90, -90)
  point P9 (-5.973324, 57)
  point P10 (5.973324, 57)
  point P11 (17.07309, 51.059023)
  point P12 (12.894904, 50.322296)
  point P13 (26.343459, 30.407302)
  point P14 (11.630844, -20)
  point P15 (0, 57.951347)
  point P16 (21.81067, 27.683727)
  dimension "d352" = 15
  dimension "d359" = 2.1
  dimension "d360" = 2.1
  dimension "d361" = 2.1
  dimension "d362" = 2.1
  dimension "d405" = 1
  dimension "d410" = 1
  dimension "d411" = 6
  dimension "d412" = 20
  dimension "d413" = 5
  dimension "d414" = 1.5
  dimension "d422" = 12
  dimension "d426" = 5
  dimension "d427" = 4
  dimension "d428" = 5
  dimension "d430" = 5
  dimension "d432" = 50
  dimension "d434" = 4
  dimension "d435" = 4
  dimension "d436" = 130
  dimension "d437" = 18
  dimension "d438" = 4
  dimension "d439" = 1.5
  dimension "d451" = 4
  dimension "d466" = 5
  dimension "d467" = 45
  dimension "d468" = 4
  dimension "d469" = 5
  dimension "d470" = 3
  dimension "d471" = 6
  dimension "d491" = 1.25
  dimension "d492" = 1.6
  dimension "d497" = 3
  dimension "d499" = 3
  dimension "d503" = 1.25
  dimension "d504" = 1.6
  dimension "d505" = 3
  dimension "d506" = 3.5
  dimension "d507" = 9
  dimension "d509" = 1.6
  dimension "d510" = 3
  dimension "d515" = 1.5
  dimension "d516" = 1.5
  dimension "d517" = 2.25
  dimension "d518" = 2.25
  dimension "d520" = 5
  dimension "d521" = 5
  dimension "d532" = 0.95
  dimension "d533" = 1.6
  dimension "d534" = 3
  dimension "d538" = 2.5
  dimension "d539" = 5
  dimension "d546" = 87.42181
  dimension "d547" = 9.5
  dimension "d548" = 13
  dimension "d549" = 56.42181
  dimension "d552" = 2
  dimension "d556" = 0.2
  dimension "d557" = 0.2
  dimension "d560" = 2.1
  constraints: 178 end point, 49 horizontal alignment, 30 centre point, 23 point on line, 21 coincident, 20 parallel, 12 equal radius, 9 perpendicular, 8 collinear, 4 midpoint, 2 horizontal, 1 equal length, 1 tangent, 1 vertical, 43 other
  measures "d352" diameter of A12
  measures "d359" diameter of A13
  measures "d360" diameter of A14
  measures "d361" diameter of A15
  measures "d362" diameter of A16
  measures "d405" distance from line of L265 L110.start
  measures "d410" distance between parallel lines of L268 L265
  measures "d411" distance of L266.end L267.start
  measures "d412" angle of L267 L265
  measures "d413" distance between parallel lines of L270 L265
  measures "d414" distance between parallel lines of L271 L100
  measures "d422" angle of L161 L272
  measures "d426" distance between parallel lines of L272 L275
  measures "d428" distance between parallel lines of L280 L238
  measures "d432" angle of L158 L237
  measures "d434" distance of L158.start L282.end
  measures "d435" distance of L158.end L284.end
  measures "d436" angle of L286 L287
  measures "d437" distance of L159.start L286.end
  measures "d438" distance of L237.end L290.start
  measures "d439" distance between parallel lines of L160 L291
  measures "d451" distance between parallel lines of L283 L281
  measures "d466" distance between parallel lines of L159 L296
  measures "d467" angle of L297 L277
  measures "d468" distance of L295.end L296.end
  measures "d469" distance between parallel lines of L302 L231
  measures "d470" distance of L301.end L302.end
  measures "d471" distance of L278.start L303.end
  measures "d491" diameter of A18
  measures "d492" diameter of A19
  measures "d497" diameter of A20
  measures "d499" distance from line of L278 A18.centre
  measures "d503" diameter of A24
  measures "d504" diameter of A25
  measures "d505" diameter of A26
  measures "d506" distance from line of L277 A24.centre
  measures "d509" diameter of A30
  measures "d510" diameter of A31
  measures "d515" distance between parallel lines of L250 L309
  measures "d516" distance between parallel lines of L311 L243
  measures "d517" distance between parallel lines of L246 L310
  measures "d518" distance between parallel lines of L308 L258
  measures "d520" distance between parallel lines of L313 L287
  measures "d521" distance between parallel lines of L161 L314
  measures "d532" diameter of A35
  measures "d533" diameter of A36
  measures "d534" diameter of A37
  measures "d538" distance from line of L161 A35.centre
  measures "d539" distance from line of L315 A35.centre
  measures "d546" distance between parallel lines of L238 L265
  measures "d547" distance between parallel lines of L310 L308
  measures "d548" distance between parallel lines of L309 L311
  measures "d549" distance of the line from the sketch origin of L265
  measures "d552" distance from line of L324 L271.start
  measures "d556" distance between parallel lines of L98 L326
  measures "d557" distance between parallel lines of L329 L102
  measures "d560" diameter of A41